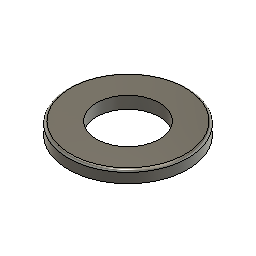
Printer stabilizer (Autodesk Fusion 360 archive; units mm, degrees)
design "Rondelle 8x15x1.5"
Autodesk Fusion 360 part; units mm, degrees
cylinder "CylindrePrimitive1" add diameter 14.95 height 1.52 placed x (1, 0, 0) y (0, 0, -1) z (0, 1, 0) at (0, 0, 0)
hole "Perçage1" at (0, 1.52, 0) direction (0, -1, 0) diameter 7.87 end through all
fillet "Congé1" radius 0.299 1 edges at (-6.9691, 1.52, 2.7031)
equation "rond_diam = 14.95 mm"
equation "tige_diam = 7.87 mm"
equation "d5 = rond_ep"
equation "rond_ep = 1.52 mm"
equation "d9 = tige_diam"
equation "d12 = rond_diam / 50"
equation "d12 = rond_diam / 50"

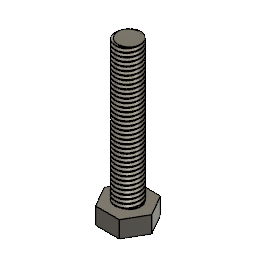
design "Vis hexa 8x50"
Autodesk Fusion 360 part; units mm, degrees
cylinder "CylindrePrimitive1" add diameter 8 height 50 placed x (1, 0, 0) y (0, 0, -1) z (0, 1, 0) at (0, 0, 0)
sketch "Esquisse3" plane through (0, 0, 0) normal (0, -1, 0) x (1, 0, 0)
  circle A0 centre (0, 0) radius 4
  line L0 (3.7528, -6.5) -> (7.5056, 0)
  line L1 (7.5056, 0) -> (3.7528, 6.5)
  line L2 (3.7528, 6.5) -> (-3.7528, 6.5)
  line L3 (-3.7528, 6.5) -> (-7.5056, 0)
  line L4 (-7.5056, 0) -> (-3.7528, -6.5)
  line L5 (-3.7528, -6.5) -> (3.7528, -6.5)
  dimension "d3" = 6.5
  constraint coincident A0.centre origin
  measures "d3" distance of A0.centre L5
extrude "Extrusion3" add sketch "Esquisse3" against normal blind 5.3
thread "Filetage2" "ISO Metric profile 8.0 M8x1.25 6g" major diameter 7.866 minor diameter 6.4455 pitch 1.25 angle 60 modelled right hand crest width 0.1833 on face at (3.9801, 20.2, -0.3983) crest through (3.933, 4.9875, 0)
equation "vis_diam = 8 mm"
equation "tete_vis_l = 13 mm"
equation "tete_vis_ep = 5.3 mm"
equation "vis_l = 50 mm"
equation "d1 = vis_l"
equation "d3 = tete_vis_l / 2"
equation "d4 = -tete_vis_ep"
